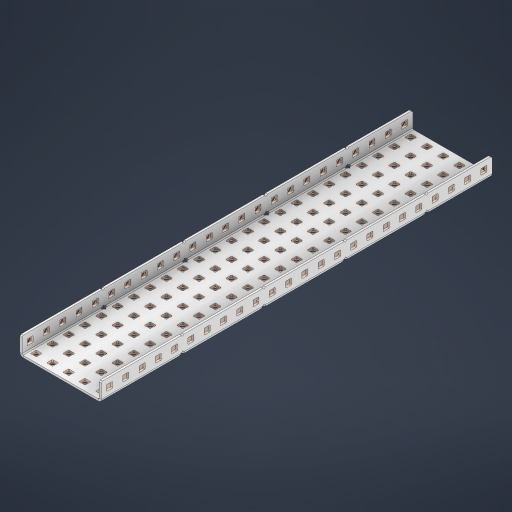
# Autodesk Inventor part: Alu C 1x3x1x35
Saved by Autodesk Inventor 2023 (Build 270158000, 158)
## iProperties
Created: 2022-07-28
Part Number: Alu C 1x3x1x35
Material: Generic
Document SubType Name: Sheet Metal
Designer: ylu12
Density: 1 g/cm^3
Sheet Metal Rule: Default
Appearance: Alu
Author: ylu12
Autodesk Inventor part; units mm, degrees
ref_plane "YZ Plane" through (0, 0, 0) normal (1, 0, 0) x (0, 1, 0)
ref_plane "XZ Plane" through (0, 0, 0) normal (0, 1, 0) x (-1, 0, 0)
ref_plane "XY Plane" through (0, 0, 0) normal (0, 0, 1) x (1, 0, 0)
sketch "Sketch1" plane through (0, 0, 0) normal (0, 1, 0) x (-1, 0, 0)
  line L0 (-31.75, 0) -> (31.75, 0)
  line L1 (31.75, 0) -> (31.75, -304.8)
  line L2 (31.75, -304.8) -> (-31.75, -304.8)
  line L3 (-31.75, -304.8) -> (-31.75, 0)
  line L4 (31.75, 0) -> (-31.75, -304.8) construction
  point P0 (0, 0)
  point P1 (0, 0)
  dimension "d0" = 63.5
  dimension "d1" = 304.8
  measures "d0" distance of L1.end L2.end
  measures "d1" distance of L0.end L1.end
extrude "Plate1" add sketch "Sketch1" along normal blind 1.5875
sketch "Sketch2" plane through (30.1625, 0, -304.8) normal (1, 0, 0) x (0, 1, 0)
  line L0 (0, 304.8) -> (0, 0)
  line L1 (0, 0) -> (14.2875, 0)
  line L2 (14.2875, 0) -> (14.2875, 304.8)
  line L3 (14.2875, 304.8) -> (0, 304.8)
  constraints: 6 end point, 1 horizontal, 1 perpendicular, 1 vertical
edge flange "Flanges" height 12.7 angle 90 thickness 1.5875 bend radius 0.7937 thickness toward (1, 0, 0) relief straight relief width 1.5875 relief depth 0.7937 corner gap 1.5875 corner form 0 edges at (31.75, 1.5875, -152.4) (-31.75, 1.5875, -152.4) wall of the first edge with corners at (30.1625, 0, 0) (30.1625, 0, -304.8) (30.1625, 14.2875, -304.8) (30.1625, 14.2875, 0)
bend "Bend1"
corner "Corner1"
sketch "Sketch3" plane through (31.75, 2.3813, -304.8) normal (1, 0, 0) x (0, 0, -1)
  line L0 (-300.2534, 7.8676) -> (-296.6466, 7.8676)
  line L1 (-296.1386, 7.3596) -> (-296.1386, 3.7528)
  line L2 (-296.6466, 3.2448) -> (-300.2534, 3.2448)
  line L3 (-300.7614, 3.7528) -> (-300.7614, 7.3596)
  arc A0 (-300.2534, 7.8676) -> (-300.7614, 7.3596) centre (-300.2534, 7.3596) ccw
  arc A1 (-296.1386, 7.3596) -> (-296.6466, 7.8676) centre (-296.6466, 7.3596) ccw
  arc A2 (-296.6466, 3.2448) -> (-296.1386, 3.7528) centre (-296.6466, 3.7528) ccw
  arc A3 (-300.7614, 3.7528) -> (-300.2534, 3.2448) centre (-300.2534, 3.7528) ccw
  line L4 (-304.8, 0) -> (-304.8, 11.9062) construction
  line L5 (-304.8, 11.9062) -> (0, 11.9063) construction
  line L6 (-300.2534, 7.3596) -> (-296.6466, 3.7528) construction
  point P0 (-304.8, -2.3813)
  point P1 (-296.1386, 3.2448)
  point P2 (-300.7614, 3.2448)
  point P3 (-298.45, 5.5562)
  dimension "d16" = 4.6228
  dimension "d17" = 0.508
  dimension "d20" = 6.35
  dimension "d21" = 6.35
  constraints: 10 end point, 8 point on circle, 8 tangent, 4 centre point, 4 point on line, 3 equal radius, 2 parallel, 2 perpendicular, 1 horizontal, 1 midpoint
  measures "d16" distance of point (-296.139, 3.245) point (-300.761, 3.245)
  measures "d17" radius of A0
  measures "d20" distance from line of point (-298.45, 5.556) L4
  measures "d21" distance from line of L5 point (-298.45, 5.556)
extrude "Flange Stamp" cut sketch "Sketch3" against normal blind 1.5875
sketch "Sketch7" plane through (31.75, 2.3813, 0) normal (1, 0, 0) x (0, 0, -1)
  arc A0 (4.5466, 7.8676) -> (4.0386, 7.3596) centre (4.5466, 7.3596) ccw construction
  arc A1 (8.1534, 3.2448) -> (8.6614, 3.7528) centre (8.1534, 3.7528) ccw construction
  circle A2 centre (6.35, 5.5563) radius 2.1844
  line L0 (4.5466, 7.3596) -> (8.1534, 3.7528) construction
  point P0 (0, -2.3812)
  dimension "d46" = 4.3688
  constraints: 2 end point, 1 centre point, 1 midpoint
  measures "d46" diameter of A2
surface extrude "Flange Circle" sketch "Sketch7" against normal up to surface (1.5875 mm away) shown yes curves A2
ref_plane "Flange Pattern Plane" through (31.75, 7.9375, -4.5466) normal (0, 1, 0) x (1, 0, 0)
pattern_sketch "Flange Pattern" of "Flange Circle", "Flange Stamp" from (31.75, 7.9375, -6.35) facing (1, 0, 0) copies at (31.75, 7.9375, -19.05) facing (1, 0, 0) at (31.75, 7.9375, -31.75) facing (1, 0, 0) at (31.75, 7.9375, -44.45) facing (1, 0, 0) at (31.75, 7.9375, -57.15) facing (1, 0, 0) at (31.75, 7.9375, -69.85) facing (1, 0, 0) at (31.75, 7.9375, -82.55) facing (1, 0, 0) at (31.75, 7.9375, -95.25) facing (1, 0, 0) at (31.75, 7.9375, -107.95) facing (1, 0, 0) at (31.75, 7.9375, -120.65) facing (1, 0, 0) at (31.75, 7.9375, -133.35) facing (1, 0, 0) at (31.75, 7.9375, -146.05) facing (1, 0, 0) at (31.75, 7.9375, -158.75) facing (1, 0, 0) at (31.75, 7.9375, -171.45) facing (1, 0, 0) at (31.75, 7.9375, -184.15) facing (1, 0, 0) at (31.75, 7.9375, -196.85) facing (1, 0, 0) at (31.75, 7.9375, -209.55) facing (1, 0, 0) at (31.75, 7.9375, -222.25) facing (1, 0, 0) at (31.75, 7.9375, -234.95) facing (1, 0, 0) at (31.75, 7.9375, -247.65) facing (1, 0, 0) at (31.75, 7.9375, -260.35) facing (1, 0, 0) at (31.75, 7.9375, -273.05) facing (1, 0, 0) at (31.75, 7.9375, -285.75) facing (1, 0, 0) at (31.75, 7.9375, -298.45) facing (1, 0, 0) at (-31.75, 7.9375, -6.35) facing (-1, 0, 0) at (-31.75, 7.9375, -19.05) facing (-1, 0, 0) at (-31.75, 7.9375, -31.75) facing (-1, 0, 0) at (-31.75, 7.9375, -44.45) facing (-1, 0, 0) at (-31.75, 7.9375, -57.15) facing (-1, 0, 0) at (-31.75, 7.9375, -69.85) facing (-1, 0, 0) at (-31.75, 7.9375, -82.55) facing (-1, 0, 0) at (-31.75, 7.9375, -95.25) facing (-1, 0, 0) at (-31.75, 7.9375, -107.95) facing (-1, 0, 0) at (-31.75, 7.9375, -120.65) facing (-1, 0, 0) at (-31.75, 7.9375, -133.35) facing (-1, 0, 0) at (-31.75, 7.9375, -146.05) facing (-1, 0, 0) at (-31.75, 7.9375, -158.75) facing (-1, 0, 0) at (-31.75, 7.9375, -171.45) facing (-1, 0, 0) at (-31.75, 7.9375, -184.15) facing (-1, 0, 0) at (-31.75, 7.9375, -196.85) facing (-1, 0, 0) at (-31.75, 7.9375, -209.55) facing (-1, 0, 0) at (-31.75, 7.9375, -222.25) facing (-1, 0, 0) at (-31.75, 7.9375, -234.95) facing (-1, 0, 0) at (-31.75, 7.9375, -247.65) facing (-1, 0, 0) at (-31.75, 7.9375, -260.35) facing (-1, 0, 0) at (-31.75, 7.9375, -273.05) facing (-1, 0, 0) at (-31.75, 7.9375, -285.75) facing (-1, 0, 0) at (-31.75, 7.9375, -298.45) facing (-1, 0, 0)
sketch "Sketch8" plane through (0, 0, 0) normal (0, -1, 0) x (1, 0, 0)
  line L0 (29.3687, 0) -> (-29.3687, 0) construction
  line L1 (27.2034, -4.0386) -> (23.5966, -4.0386)
  line L2 (23.0886, -4.5466) -> (23.0886, -8.1534)
  line L3 (23.5966, -8.6614) -> (27.2034, -8.6614)
  line L4 (27.7114, -8.1534) -> (27.7114, -4.5466)
  arc A0 (27.7114, -4.5466) -> (27.2034, -4.0386) centre (27.2034, -4.5466) ccw
  arc A1 (27.2034, -8.6614) -> (27.7114, -8.1534) centre (27.2034, -8.1534) ccw
  arc A2 (23.0886, -8.1534) -> (23.5966, -8.6614) centre (23.5966, -8.1534) ccw
  arc A3 (23.5966, -4.0386) -> (23.0886, -4.5466) centre (23.5966, -4.5466) ccw
  line L5 (27.2034, -4.5466) -> (23.5966, -8.1534) construction
  line L6 (31.75, 0) -> (31.75, -304.8) construction
  point P0 (0, 0)
  point P1 (23.0886, -8.6614)
  point P2 (27.7114, -8.6614)
  point P3 (25.4, -6.35)
  dimension "d49" = 4.6228
  dimension "d50" = 0.508
  dimension "d51" = 6.35
  dimension "d52" = 6.35
  constraints: 10 end point, 8 point on circle, 8 tangent, 4 centre point, 4 point on line, 3 equal radius, 2 parallel, 2 perpendicular, 1 horizontal, 1 midpoint
  measures "d49" distance of point (27.711, -8.661) point (23.089, -8.661)
  measures "d50" radius of A0
  measures "d51" distance from line of L6 point (25.4, -6.35)
  measures "d52" distance from line of L0 point (25.4, -6.35)
extrude "Body Stamp" cut sketch "Sketch8" against normal blind 1.5875
sketch "Sketch9" plane through (0, 0, 0) normal (0, -1, 0) x (1, 0, 0)
  arc A0 (27.7114, -4.5466) -> (27.2034, -4.0386) centre (27.2034, -4.5466) ccw construction
  arc A1 (23.0886, -8.1534) -> (23.5966, -8.6614) centre (23.5966, -8.1534) ccw construction
  line L0 (27.2034, -4.5466) -> (23.5966, -8.1534) construction
  circle A2 centre (25.4, -6.35) radius 2.1844
  point P0 (0, 0)
  dimension "d55" = 4.3688
  constraints: 2 end point, 1 centre point, 1 midpoint
  measures "d55" diameter of A2
surface extrude "Body Circle" sketch "Sketch9" against normal up to surface (1.5875 mm away) shown yes curves A2
pattern_sketch "Body Pattern" of "Body Stamp", "Body Circle" from (25.4, 0, -6.35) copies at (25.4, 0, -19.05) at (25.4, 0, -31.75) at (25.4, 0, -44.45) at (25.4, 0, -57.15) at (25.4, 0, -69.85) at (25.4, 0, -82.55) at (25.4, 0, -95.25) at (25.4, 0, -107.95) at (25.4, 0, -120.65) at (25.4, 0, -133.35) at (25.4, 0, -146.05) at (25.4, 0, -158.75) at (25.4, 0, -171.45) at (25.4, 0, -184.15) at (25.4, 0, -196.85) at (25.4, 0, -209.55) at (25.4, 0, -222.25) at (25.4, 0, -234.95) at (25.4, 0, -247.65) at (25.4, 0, -260.35) at (25.4, 0, -273.05) at (25.4, 0, -285.75) at (25.4, 0, -298.45) at (12.7, 0, -6.35) at (12.7, 0, -19.05) at (12.7, 0, -31.75) at (12.7, 0, -44.45) at (12.7, 0, -57.15) at (12.7, 0, -69.85) at (12.7, 0, -82.55) at (12.7, 0, -95.25) at (12.7, 0, -107.95) at (12.7, 0, -120.65) at (12.7, 0, -133.35) at (12.7, 0, -146.05) at (12.7, 0, -158.75) at (12.7, 0, -171.45) at (12.7, 0, -184.15) at (12.7, 0, -196.85) at (12.7, 0, -209.55) at (12.7, 0, -222.25) at (12.7, 0, -234.95) at (12.7, 0, -247.65) at (12.7, 0, -260.35) at (12.7, 0, -273.05) at (12.7, 0, -285.75) at (12.7, 0, -298.45) at (0, 0, -6.35) at (0, 0, -19.05) at (0, 0, -31.75) at (0, 0, -44.45) at (0, 0, -57.15) at (0, 0, -69.85) at (0, 0, -82.55) at (0, 0, -95.25) at (0, 0, -107.95) at (0, 0, -120.65) at (0, 0, -133.35) at (0, 0, -146.05) at (0, 0, -158.75) at (0, 0, -171.45) at (0, 0, -184.15) at (0, 0, -196.85) at (0, 0, -209.55) at (0, 0, -222.25) at (0, 0, -234.95) at (0, 0, -247.65) at (0, 0, -260.35) at (0, 0, -273.05) at (0, 0, -285.75) at (0, 0, -298.45) at (-12.7, 0, -6.35) at (-12.7, 0, -19.05) at (-12.7, 0, -31.75) at (-12.7, 0, -44.45) at (-12.7, 0, -57.15) at (-12.7, 0, -69.85) at (-12.7, 0, -82.55) at (-12.7, 0, -95.25) at (-12.7, 0, -107.95) at (-12.7, 0, -120.65) at (-12.7, 0, -133.35) at (-12.7, 0, -146.05) at (-12.7, 0, -158.75) at (-12.7, 0, -171.45) at (-12.7, 0, -184.15) at (-12.7, 0, -196.85) at (-12.7, 0, -209.55) at (-12.7, 0, -222.25) at (-12.7, 0, -234.95) at (-12.7, 0, -247.65) at (-12.7, 0, -260.35) at (-12.7, 0, -273.05) at (-12.7, 0, -285.75) at (-12.7, 0, -298.45) at (-25.4, 0, -6.35) at (-25.4, 0, -19.05) at (-25.4, 0, -31.75) at (-25.4, 0, -44.45) at (-25.4, 0, -57.15) at (-25.4, 0, -69.85) at (-25.4, 0, -82.55) at (-25.4, 0, -95.25) at (-25.4, 0, -107.95) at (-25.4, 0, -120.65) at (-25.4, 0, -133.35) at (-25.4, 0, -146.05) at (-25.4, 0, -158.75) at (-25.4, 0, -171.45) at (-25.4, 0, -184.15) at (-25.4, 0, -196.85) at (-25.4, 0, -209.55) at (-25.4, 0, -222.25) at (-25.4, 0, -234.95) at (-25.4, 0, -247.65) at (-25.4, 0, -260.35) at (-25.4, 0, -273.05) at (-25.4, 0, -285.75) at (-25.4, 0, -298.45)
sketch "Arc Length" plane through (30.1625, 2.3813, 0) normal (0, 0, 1) x (1, 0, 0)
  line L0 (0, 0) -> (1.5875, 0) construction
  arc A0 (-0.7937, -0.7937) -> (0, 0) centre (-0.7937, 0) ccw construction
  line L1 (-0.7937, -2.3812) -> (-0.7937, -0.7937) construction
  arc A1 (-0.7937, -2.3812) -> (1.5875, 0) centre (-0.7937, 0) ccw construction
  point P0 (-30.1625, -2.3812)
  dimension "d85" = 3.7405
  dimension "d92" = 1.2468
sketch "Sketch13" plane through (31.75, 14.2875, 0) normal (1, 0, 0) x (0, 0, -1)
  line L0 (0, 0) -> (304.8, 0) construction
  line L1 (62.4078, 0) -> (63.4238, -1.016)
  line L2 (63.4238, -1.016) -> (64.4398, 0)
  line L3 (62.4078, 0) -> (64.4398, 0)
  line L4 (304.8, -11.9063) -> (0, -11.9062) construction
  line L5 (63.4238, -10.8903) -> (61.161, -13.1531)
  line L6 (61.161, -13.1531) -> (63.4238, -15.4159)
  line L7 (63.4238, -15.4159) -> (65.6866, -13.1531)
  line L8 (65.6866, -13.1531) -> (63.4238, -10.8903)
  line L9 (63.4238, -10.8903) -> (63.4238, -15.4159) construction
  line L10 (63.4238, -1.016) -> (63.4238, -10.8903) construction
  line L11 (0, -11.9062) -> (304.8, -11.9063) construction
  point P0 (0, -14.2875)
  dimension "d86" = 4.5256
  dimension "d88" = 1.016
  dimension "d91" = 1.016
  dimension "d102" = 63.4238
  constraints: 19 end point, 6 perpendicular, 2 point on line, 2 vertical, 1 collinear
  measures "d86" distance of L5.start L6.end
  measures "d88" distance from line of L0 L1.end
  measures "d91" distance from line of L5.start L11
  measures "d102" distance from line of L0.start L10
cut across bends "Notch" sketch "Sketch13" k factor 0.44
mirror "Notch Mirror" about plane through (0, 0, 0) normal (1, 0, 0) of "Notch"
pattern_linear "Notch Pattern" count 4 spacing 63.5 along (0, 0, -1) of "Notch", "Notch Mirror"
chamfer "End Chamfer" distance 1.016 angle 45 4 edges at (-30.9562, 14.2875, 0) (30.9562, 14.2875, 0) (-30.9562, 14.2875, -304.8) (30.9563, 14.2875, -304.8)
sketch "Sketch14" plane through (-31.75, 2.3812, 139.7) normal (1, 0, 0) x (0, 0, -1)
  line L0 (139.7, 11.9063) -> (444.5, 11.9063) construction
  line L1 (139.7, 0) -> (139.7, 11.9063) construction
  line L2 (139.7, -2.3813) -> (444.5, -2.3813) construction
  line L3 (139.7, 11.9063) -> (444.5, 11.9063)
  line L4 (444.5, 11.9063) -> (444.5, -2.3813)
  line L5 (444.5, -2.3813) -> (139.7, -2.3813)
  line L6 (139.7, -2.3813) -> (139.7, 11.9063)
  point P0 (139.7, -2.3812)
  point P1 (382.0521, -1.9844)
  constraints: 8 end point, 2 collinear, 2 parallel, 1 horizontal, 1 perpendicular, 1 other
extrude "Half Cut" [suppressed]
sketch "Flange Pattern Sketch" plane through (31.75, 7.9375, -4.5466) normal (0, 1, 0) x (1, 0, 0)
  line L0 (0, 3.6068) -> (0, 0) construction
  line L1 (-76.2986, -4.5466) -> (13.2918, -4.5466) construction
  line L2 (0, 0) -> (-1.5875, 0) construction
  point P0 (-31.75, -4.5466)
  point P1 (0, 1.8034)
  point P2 (0, 14.5034)
  point P3 (0, 27.2034)
  point P4 (0, 39.9034)
  point P5 (0, 52.6034)
  point P6 (0, 65.3034)
  point P7 (0, 78.0034)
  point P8 (0, 90.7034)
  point P9 (0, 103.4034)
  point P10 (0, 116.1034)
  point P11 (0, 128.8034)
  point P12 (0, 141.5034)
  point P13 (0, 154.2034)
  point P14 (0, 166.9034)
  point P15 (0, 179.6034)
  point P16 (0, 192.3034)
  point P17 (0, 205.0034)
  point P18 (0, 217.7034)
  point P19 (0, 230.4034)
  point P20 (0, 243.1034)
  point P21 (0, 255.8034)
  point P22 (0, 268.5034)
  point P23 (0, 281.2034)
  point P24 (0, 293.9034)
  point P25 (-63.5, 1.8034)
  point P26 (-63.5, 14.5034)
  point P27 (-63.5, 27.2034)
  point P28 (-63.5, 39.9034)
  point P29 (-63.5, 52.6034)
  point P30 (-63.5, 65.3034)
  point P31 (-63.5, 78.0034)
  point P32 (-63.5, 90.7034)
  point P33 (-63.5, 103.4034)
  point P34 (-63.5, 116.1034)
  point P35 (-63.5, 128.8034)
  point P36 (-63.5, 141.5034)
  point P37 (-63.5, 154.2034)
  point P38 (-63.5, 166.9034)
  point P39 (-63.5, 179.6034)
  point P40 (-63.5, 192.3034)
  point P41 (-63.5, 205.0034)
  point P42 (-63.5, 217.7034)
  point P43 (-63.5, 230.4034)
  point P44 (-63.5, 243.1034)
  point P45 (-63.5, 255.8034)
  point P46 (-63.5, 268.5034)
  point P47 (-63.5, 281.2034)
  point P48 (-63.5, 293.9034)
  dimension "d131" = 63.5
  dimension "d134" = 12.7
  constraints: 1 horizontal, 1 midpoint, 1 vertical, 47 other
  measures "d134" distance of point (0, 1.803) point (0, 14.503)
sketch "Body Pattern Sketch" plane through (0, 0, 0) normal (0, -1, 0) x (1, 0, 0)
  line L0 (29.3687, 0) -> (-29.3687, 0) construction
  line L1 (31.75, 0) -> (31.75, -304.8) construction
  circle A0 centre (25.4, -6.35) radius 2.1844 construction
  point P0 (0, 0)
  point P1 (25.4, -19.05)
  point P2 (25.4, -31.75)
  point P3 (25.4, -44.45)
  point P4 (25.4, -57.15)
  point P5 (25.4, -69.85)
  point P6 (25.4, -82.55)
  point P7 (25.4, -95.25)
  point P8 (25.4, -107.95)
  point P9 (25.4, -120.65)
  point P10 (25.4, -133.35)
  point P11 (25.4, -146.05)
  point P12 (25.4, -158.75)
  point P13 (25.4, -171.45)
  point P14 (25.4, -184.15)
  point P15 (25.4, -196.85)
  point P16 (25.4, -209.55)
  point P17 (25.4, -222.25)
  point P18 (25.4, -234.95)
  point P19 (25.4, -247.65)
  point P20 (25.4, -260.35)
  point P21 (25.4, -273.05)
  point P22 (25.4, -285.75)
  point P23 (25.4, -298.45)
  point P24 (12.7, -6.35)
  point P25 (12.7, -19.05)
  point P26 (12.7, -31.75)
  point P27 (12.7, -44.45)
  point P28 (12.7, -57.15)
  point P29 (12.7, -69.85)
  point P30 (12.7, -82.55)
  point P31 (12.7, -95.25)
  point P32 (12.7, -107.95)
  point P33 (12.7, -120.65)
  point P34 (12.7, -133.35)
  point P35 (12.7, -146.05)
  point P36 (12.7, -158.75)
  point P37 (12.7, -171.45)
  point P38 (12.7, -184.15)
  point P39 (12.7, -196.85)
  point P40 (12.7, -209.55)
  point P41 (12.7, -222.25)
  point P42 (12.7, -234.95)
  point P43 (12.7, -247.65)
  point P44 (12.7, -260.35)
  point P45 (12.7, -273.05)
  point P46 (12.7, -285.75)
  point P47 (12.7, -298.45)
  point P48 (0, -6.35)
  point P49 (0, -19.05)
  point P50 (0, -31.75)
  point P51 (0, -44.45)
  point P52 (0, -57.15)
  point P53 (0, -69.85)
  point P54 (0, -82.55)
  point P55 (0, -95.25)
  point P56 (0, -107.95)
  point P57 (0, -120.65)
  point P58 (0, -133.35)
  point P59 (0, -146.05)
  point P60 (0, -158.75)
  point P61 (0, -171.45)
  point P62 (0, -184.15)
  point P63 (0, -196.85)
  point P64 (0, -209.55)
  point P65 (0, -222.25)
  point P66 (0, -234.95)
  point P67 (0, -247.65)
  point P68 (0, -260.35)
  point P69 (0, -273.05)
  point P70 (0, -285.75)
  point P71 (0, -298.45)
  point P72 (-12.7, -6.35)
  point P73 (-12.7, -19.05)
  point P74 (-12.7, -31.75)
  point P75 (-12.7, -44.45)
  point P76 (-12.7, -57.15)
  point P77 (-12.7, -69.85)
  point P78 (-12.7, -82.55)
  point P79 (-12.7, -95.25)
  point P80 (-12.7, -107.95)
  point P81 (-12.7, -120.65)
  point P82 (-12.7, -133.35)
  point P83 (-12.7, -146.05)
  point P84 (-12.7, -158.75)
  point P85 (-12.7, -171.45)
  point P86 (-12.7, -184.15)
  point P87 (-12.7, -196.85)
  point P88 (-12.7, -209.55)
  point P89 (-12.7, -222.25)
  point P90 (-12.7, -234.95)
  point P91 (-12.7, -247.65)
  point P92 (-12.7, -260.35)
  point P93 (-12.7, -273.05)
  point P94 (-12.7, -285.75)
  point P95 (-12.7, -298.45)
  point P96 (-25.4, -6.35)
  point P97 (-25.4, -19.05)
  point P98 (-25.4, -31.75)
  point P99 (-25.4, -44.45)
  point P100 (-25.4, -57.15)
  point P101 (-25.4, -69.85)
  point P102 (-25.4, -82.55)
  point P103 (-25.4, -95.25)
  point P104 (-25.4, -107.95)
  point P105 (-25.4, -120.65)
  point P106 (-25.4, -133.35)
  point P107 (-25.4, -146.05)
  point P108 (-25.4, -158.75)
  point P109 (-25.4, -171.45)
  point P110 (-25.4, -184.15)
  point P111 (-25.4, -196.85)
  point P112 (-25.4, -209.55)
  point P113 (-25.4, -222.25)
  point P114 (-25.4, -234.95)
  point P115 (-25.4, -247.65)
  point P116 (-25.4, -260.35)
  point P117 (-25.4, -273.05)
  point P118 (-25.4, -285.75)
  point P119 (-25.4, -298.45)
  dimension "d62" = 12.7
  dimension "d65" = 12.7
  dimension "d139" = 12.7
  constraints: 1 coincident, 1 horizontal, 1 vertical, 119 other
  measures "d139" distance of point (25.4, -19.05) point (25.4, -6.35)
equation "\"d1\" = 12.7 * Length"
equation "\"d18\" = Thickness"
equation "\"d53\" = Thickness"
equation "\"d89\" = Thickness"
equation "\"d2\" = Thickness"
equation "\"d3\" = BendReliefWidth"
equation "\"d4\" = BendReliefDepth"
equation "\"d5\" = MinimumRemnant"
equation "\"d6\" = TransitionRadius"
equation "\"d10\" = CornerReliefSize"
equation "\"d11\" = GapSize"
equation "\"d12\" = JacobiRadiusSize"
equation "\"BendRadius\" = Thickness"
equation "\"BendReliefWidth\" = Thickness"
equation "\"BendReliefDepth\" = 0.5 * Thickness"
equation "\"CornerReliefSize\" = 4 * Thickness"
equation "\"MinimumRemnant\" = 2 * Thickness"
equation "\"TransitionRadius\" = BendRadius"
equation "\"JacobiRadiusSize\" = BendRadius"
equation "\"GapSize\" = Thickness"
equation "\"Length\" = 24"
equation "\"Thickness\" = 1.5875"
body "Solid1"
body "Srf1"
body "Srf2"
body "Srf91"
body "Srf92"
body "Srf856"
body "Srf1310"
body "Srf1311"
body "Srf1312"
body "Srf1376"
body "Srf1377"
body "Srf1728"
body "Srf1755"
body "Srf1878"
body "Srf1879"
body "Srf1880"
body "Srf1881"
body "Srf1882"
body "Srf1883"
body "Srf1884"
body "Srf1885"
body "Srf1886"
body "Srf1887"
body "Srf1888"
body "Srf1889"
body "Srf1890"
body "Srf1891"
body "Srf1892"
body "Srf1893"
body "Srf1894"
body "Srf1895"
body "Srf1896"
body "Srf1897"
body "Srf1898"
body "Srf1899"
body "Srf1900"
body "Srf1901"
body "Srf1902"
body "Srf1903"
body "Srf1904"
body "Srf1905"
body "Srf1906"
body "Srf1942"
body "Srf1943"
body "Srf1944"
body "Srf1945"
body "Srf1946"
body "Srf1947"
body "Srf1948"
body "Srf1949"
body "Srf1950"
body "Srf1951"
body "Srf1952"
body "Srf1953"
body "Srf1954"
body "Srf1955"
body "Srf1956"
body "Srf1957"
body "Srf1958"
body "Srf1959"
body "Srf1960"
body "Srf1961"
body "Srf1962"
body "Srf1963"
body "Srf1964"
body "Srf1965"
body "Srf1966"
body "Srf1967"
body "Srf1968"
body "Srf1969"
body "Srf1970"
body "Srf2111"
body "Srf2112"
body "Srf2113"
body "Srf2114"
body "Srf2115"
body "Srf2116"
body "Srf2117"
body "Srf2118"
body "Srf2119"
body "Srf2120"
body "Srf2121"
body "Srf2122"
body "Srf2123"
body "Srf2146"
body "Srf2147"
body "Srf2148"
body "Srf2149"
body "Srf2150"
body "Srf2151"
body "Srf2152"
body "Srf2153"
body "Srf2154"
body "Srf2155"
body "Srf2156"
body "Srf2157"
body "Srf2158"
body "Srf2159"
body "Srf2160"
body "Srf2161"
body "Srf2162"
body "Srf2163"
body "Srf2164"
body "Srf2165"
body "Srf2166"
body "Srf2167"
body "Srf2168"
body "Srf2169"
body "Srf2170"
body "Srf2171"
body "Srf2172"
body "Srf2173"
body "Srf2174"
body "Srf2175"
body "Srf2176"
body "Srf2177"
body "Srf2178"
body "Srf2179"
body "Srf2180"
body "Srf2181"
body "Srf2182"
body "Srf2183"
body "Srf2184" dims "d2" = 1.5875 (= Thickness), "d10" = 6.35 (= CornerReliefSize)
body "Srf2185"
body "Srf2186"
body "Srf2187"
body "Srf2188"
body "Srf2189"
body "Srf2190"
body "Srf2191"
body "Srf2192"
body "Srf2193"
body "Srf2194"
body "Srf2195"
body "Srf2196"
body "Srf2197"
body "Srf2198"
body "Srf2199"
body "Srf2200"
body "Srf2201"
body "Srf2202"
body "Srf2203"
body "Srf2204"
body "Srf2205"
body "Srf2206"
body "Srf2207"
body "Srf2208"
body "Srf2209"
body "Srf2210"
body "Srf2211"
body "Srf2212"
body "Srf2213"
body "Srf2214"
body "Srf2215"
body "Srf2216"
body "Srf2217"
body "Srf2218"
body "Srf2219"
body "Srf2220"
body "Srf2221"
body "Srf2222"
body "Srf2223"
body "Srf2224"
body "Srf2225"
body "Srf2226"
body "Srf2227"
body "Srf2228"
body "Srf2229"
body "Srf2230"
